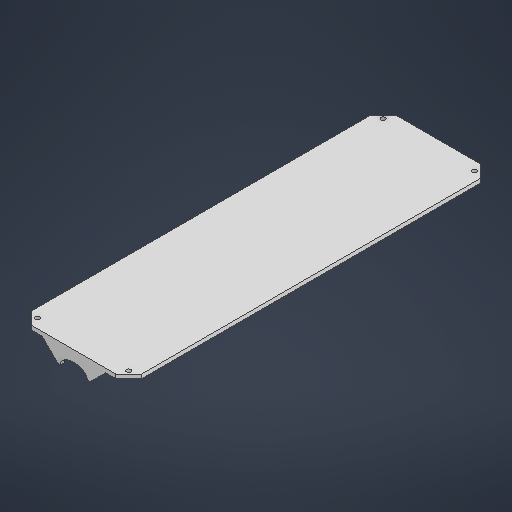
# Autodesk Inventor part: DriverFestingToppur
Saved by Autodesk Inventor 2026.1 (Build 301233000, 233)
## iProperties
Created: 2026-01-13
Part Number: DriverFestingToppur
Material: Generic
Document SubType Name: Modeling
Designer: Brynjar
Density: 1 g/cm^3
Appearance: Default
Author: Brynjar
Autodesk Inventor part; units mm, degrees
ref_plane "YZ Plane" through (0, 0, 0) normal (1, 0, 0) x (0, 1, 0)
ref_plane "XY Plane" through (0, 0, 0) normal (0, 0, 1) x (1, 0, 0)
derived "DriverFesting.ipt"
sketch "Sketch1" plane through (0, 0, 0) normal (0, 1, 0) x (-1, 0, 0)
  line L0 (-15, -136) -> (-66, -136) construction
  line L1 (-78, -148) -> (-78, -254) construction
  line L2 (-66, -266) -> (-15, -266) construction
  line L3 (-3, -254) -> (-3, -148) construction
  line L4 (-15, -133) -> (-66, -133) construction
  line L5 (-78, -121) -> (-78, -15) construction
  line L6 (-66, -3) -> (-15, -3) construction
  line L7 (-3, -15) -> (-3, -121) construction
  line L8 (-78, -136) -> (-78, -133) construction
  line L9 (-9.5147, 0) -> (-71.4853, 0)
  line L10 (-81, -9.5147) -> (-81, -259.4853)
  line L11 (-71.4853, -269) -> (-9.5147, -269)
  line L12 (0, -259.4853) -> (0, -9.5147)
  line L13 (-3, -3) -> (0, -3) construction
  line L14 (-3, -3) -> (-3, 0) construction
  line L15 (-78, -266) -> (-78, -269) construction
  line L16 (-78, -266) -> (-81, -266) construction
  line L17 (-3, -201) -> (-78, -201) construction
  line L18 (-23, -142.5) -> (-58, -142.5) construction
  line L19 (-58, -142.5) -> (-58, -259.5) construction
  line L20 (-58, -259.5) -> (-23, -259.5) construction
  line L21 (-23, -259.5) -> (-23, -142.5) construction
  line L22 (-23, -142.5) -> (-58, -259.5) construction
  line L23 (-58, -142.5) -> (-23, -259.5) construction
  circle A0 centre (-23, -259.5) radius 2.5 construction
  circle A1 centre (-58, -259.5) radius 2.5 construction
  circle A2 centre (-58, -142.5) radius 2.5 construction
  circle A3 centre (-23, -142.5) radius 2.5 construction
  line L24 (-15, -266) -> (-3, -254) construction
  line L25 (-66, -266) -> (-78, -254) construction
  line L26 (-3, -148) -> (-15, -136) construction
  line L27 (-66, -136) -> (-78, -148) construction
  line L28 (-15, -133) -> (-3, -121) construction
  line L29 (-66, -133) -> (-78, -121) construction
  line L30 (-3, -15) -> (-15, -3) construction
  line L31 (-66, -3) -> (-78, -15) construction
  line L32 (0, -259.4853) -> (-9.5147, -269)
  line L33 (-81, -259.4853) -> (-71.4853, -269)
  line L34 (-71.4853, 0) -> (-81, -9.5147)
  line L35 (0, -9.5147) -> (-9.5147, 0)
  line L36 (-4.7574, -264.2426) -> (-9, -260) construction
  circle A4 centre (-6.8345, -134.5) radius 2.5 construction
  circle A5 centre (-74.1655, -134.5) radius 2.5 construction
  circle A6 centre (-6.8345, -134.5) radius 6.8345 construction
  circle A7 centre (-74.1655, -134.5) radius 6.8345 construction
  circle A8 centre (-6.8345, -134.5) radius 5.25 construction
  circle A9 centre (-74.1655, -134.5) radius 5.25 construction
  line L37 (-4.7574, -4.7574) -> (-9, -9) construction
  circle A10 centre (-6.8787, -6.8787) radius 1.6
  line L38 (-76.2426, -4.7574) -> (-72, -9) construction
  line L39 (-76.2426, -264.2426) -> (-72, -260) construction
  circle A11 centre (-74.1213, -6.8787) radius 1.6
  circle A12 centre (-74.1213, -262.1213) radius 1.6
  circle A13 centre (-6.8787, -262.1213) radius 1.6
  point P0 (0, 0)
  point P1 (-3, -136)
  point P2 (-3, -266)
  point P3 (-3, -133)
  point P4 (-78, -3)
  point P5 (-81, -269)
  point P6 (-81, 0)
  point P7 (0, -269)
  point P8 (-40.5, -201)
  dimension "d7" = 3.2
  measures "d7" diameter of A10
ref_plane "Work Plane1" through (40.5, 41, 0) normal (0, 1, 0) x (-1, 0, 0)
sketch "Sketch3" plane through (40.5, 41, 0) normal (0, 1, 0) x (-1, 0, 0)
  line L0 (-37.5, -266) -> (-37.5, -269) construction
  circle A0 centre (-33.6213, -262.1213) radius 1.6 projected
  line L1 (-35.7426, -264.2426) -> (-31.5, -260) construction
  line L2 (-25.5, -266) -> (-37.5, -254) construction
  line L3 (-37.5, -266) -> (-40.5, -266) construction
  line L4 (-40.5, -259.4853) -> (-30.9853, -269) projected
  circle A1 centre (-17.5, -259.5) radius 2.5 construction
  line L5 (-25.5, -266) -> (25.5, -266) construction
  line L6 (-30.9853, -269) -> (30.9853, -269) projected
  line L7 (-17.5, -259.5) -> (17.5, -259.5) construction
  circle A2 centre (17.5, -259.5) radius 2.5 construction
  line L8 (37.5, -201) -> (-37.5, -201) construction
  circle A3 centre (33.6213, -262.1213) radius 1.6 projected
  line L9 (35.7426, -264.2426) -> (31.5, -260) construction
  line L10 (25.5, -266) -> (37.5, -254) construction
  line L11 (40.5, -259.4853) -> (30.9853, -269) projected
  line L12 (25.5, -136) -> (-25.5, -136) construction
  line L13 (-37.5, -148) -> (-37.5, -254) construction
  line L14 (37.5, -254) -> (37.5, -148) construction
  line L15 (25.5, -133) -> (-25.5, -133) construction
  line L16 (-37.5, -121) -> (-37.5, -15) construction
  line L17 (37.5, -15) -> (37.5, -121) construction
  line L18 (-37.5, -136) -> (-37.5, -133) construction
  line L19 (-40.5, -9.5147) -> (-40.5, -259.4853) projected
  line L20 (40.5, -259.4853) -> (40.5, -9.5147) projected
  line L21 (-17.5, -142.5) -> (-17.5, -259.5) construction
  line L22 (17.5, -259.5) -> (17.5, -142.5) construction
  line L23 (17.5, -142.5) -> (-17.5, -259.5) construction
  line L24 (-17.5, -142.5) -> (17.5, -259.5) construction
  line L25 (17.5, -142.5) -> (-17.5, -142.5) construction
  circle A4 centre (33.6655, -134.5) radius 2.5 construction
  circle A5 centre (33.6655, -134.5) radius 5.25 construction
  circle A6 centre (33.6655, -134.5) radius 6.8345 construction
  circle A7 centre (-17.5, -142.5) radius 2.5 construction
  circle A8 centre (17.5, -142.5) radius 2.5 construction
  line L26 (37.5, -148) -> (25.5, -136) construction
  line L27 (25.5, -133) -> (37.5, -121) construction
  line L28 (-25.5, -136) -> (-37.5, -148) construction
  circle A9 centre (-33.6655, -134.5) radius 2.5 construction
  circle A10 centre (-33.6655, -134.5) radius 5.25 construction
  circle A11 centre (-33.6655, -134.5) radius 6.8345 construction
  line L29 (-25.5, -133) -> (-37.5, -121) construction
  line L30 (-25.5, -3) -> (25.5, -3) construction
  line L31 (30.9853, 0) -> (-30.9853, 0) projected
  line L32 (37.5, -3) -> (40.5, -3) construction
  line L33 (37.5, -3) -> (37.5, 0) construction
  line L34 (37.5, -15) -> (25.5, -3) construction
  line L35 (-25.5, -3) -> (-37.5, -15) construction
  circle A12 centre (-33.6213, -6.8787) radius 1.6 projected
  line L36 (-35.7426, -4.7574) -> (-31.5, -9) construction
  line L37 (-30.9853, 0) -> (-40.5, -9.5147) projected
  line L38 (35.7426, -4.7574) -> (31.5, -9) construction
  circle A13 centre (33.6213, -6.8787) radius 1.6 projected
  line L39 (40.5, -9.5147) -> (30.9853, 0) projected
  line L40 (9.8462, 0) -> (-9.8462, 0) projected
  line L41 (0, 0) -> (-9.8462, 0) construction
  line L42 (23.5, 0) -> (11.8462, 0) projected
  line L43 (11.8462, 0) -> (9.8462, 0) projected
  line L44 (-23.5, 0) -> (-11.8462, 0) projected
  line L45 (-11.8462, 0) -> (-9.8462, 0) projected
  line L46 (25.5, 0) -> (23.5, 0) projected
  line L47 (-25.5, 0) -> (-23.5, 0) projected
  line L48 (23.5, 0) -> (-23.5, 0) projected
  point P0 (40.5, 0)
  point P1 (-40.5, -269)
  point P2 (37.5, -266)
  point P3 (40.5, -269)
  point P4 (37.5, -136)
  point P5 (37.5, -133)
  point P6 (0, -201)
  point P7 (40.5, 0)
  point P8 (-37.5, -3)
  point P9 (-40.5, 0)
  point P10 (40.5, 0)
  point P11 (0, 0)
  point P12 (0, 0)
  constraints: 3 other
extrude "Extrusion4" add sketch "Sketch3" along normal blind 3
sketch "Sketch7" plane through (9.5147, -5, 0) normal (0, 0, 1) x (1, 0, 0)
  ellipse E0 centre (30.9853, 34.5) end of major axis (40.8314, 34.5) minor radius 6.5 projected
  line L0 (30.9853, 34.5) -> (40.8314, 34.5) construction
  line L1 (30.9853, 34.5) -> (30.9853, 41) construction
  line L2 (30.9853, 46) -> (30.9853, 41) construction
  line L3 (5.4853, 5) -> (5.4853, 46) construction
  line L4 (56.4853, 5) -> (56.4853, 46) construction
  line L5 (7.4853, 46) -> (19.1391, 34.5) projected
  line L6 (19.1391, 34.5) -> (21.1391, 34.5) projected
  line L7 (54.4853, 46) -> (42.8314, 34.5) projected
  line L8 (42.8314, 34.5) -> (40.8314, 34.5) projected
  line L9 (5.4853, 46) -> (7.4853, 46) projected
  line L10 (56.4853, 46) -> (54.4853, 46) projected
  line L11 (7.4853, 46) -> (54.4853, 46) projected
  point P0 (-9.5147, 5)
  constraints: 1 other
extrude "Extrusion5" add sketch "Sketch7" against normal blind 3 contours E0 L6 L5 L11 L7 L8
body "Solid3"
